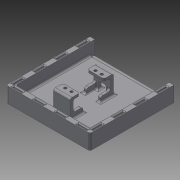
# Autodesk Inventor part: base_bottombuttonsBox
Saved by Autodesk Inventor 2014 (Build 180170000, 170)
## iProperties
Created: 2014-04-22
Part Number: base_bottombuttonsBox
Material: Generic
Document SubType Name: Modeling
Designer: t_emanb
Density: 1 g/cm^3
Appearance: Default
Author: t_emanb
Autodesk Inventor part; units mm, degrees
ref_plane "YZ Plane" through (0, 0, 0) normal (1, 0, 0) x (0, 1, 0)
ref_plane "XZ Plane" through (0, 0, 0) normal (0, 1, 0) x (-1, 0, 0)
ref_plane "XY Plane" through (0, 0, 0) normal (0, 0, 1) x (1, 0, 0)
sketch "Sketch1" plane through (0, 0, 0) normal (0, 1, 0) x (-1, 0, 0)
  line L0 (0, 0) -> (133.35, 0)
  line L1 (133.35, 0) -> (133.35, 133.35)
  line L2 (133.35, 133.35) -> (0, 133.35)
  line L3 (0, 133.35) -> (0, 0)
  dimension "d0" = 133.35
  dimension "d1" = 133.35
  constraints: 8 end point, 2 parallel, 1 horizontal, 1 perpendicular
  measures "d0" distance of L2.end L0.start
  measures "d1" distance of L0.start L0.end
extrude "Extrusion1" add sketch "Sketch1" along normal blind 5.08
sketch "Sketch2" plane through (0, 5.08, 0) normal (0, 1, 0) x (1, 0, 0)
  line L0 (0, 0) -> (-133.35, 0) projected
  line L1 (-133.35, 0) -> (-133.35, -133.35) projected
  line L2 (-133.35, -133.35) -> (0, -133.35) projected
  line L3 (0, -133.35) -> (0, 0) projected
  line L4 (-7.62, 0) -> (-7.62, -125.73)
  line L5 (-7.62, -125.73) -> (-125.73, -125.73)
  line L6 (-125.73, -125.73) -> (-125.73, 0)
  dimension "d4" = 7.62
  dimension "d5" = 7.62
  dimension "d6" = 7.62
  constraints: 6 end point, 2 point on line
  measures "d4" distance between parallel lines of L3 L4
  measures "d5" distance between parallel lines of L2 L5
  measures "d6" distance between parallel lines of L1 L6
extrude "Extrusion2" add sketch "Sketch2" along normal blind 19.05 contours L3 L2 L1 L0 L6 L5 L4
sketch "Sketch3" plane through (0, 24.13, 0) normal (0, 1, 0) x (1, 0, 0)
  line L0 (-7.62, -125.73) -> (-125.73, -125.73) projected
  line L1 (-125.73, -125.73) -> (-125.73, 0) projected
  line L2 (-133.35, 0) -> (-133.35, -133.35) projected
  line L3 (-133.35, -133.35) -> (0, -133.35) projected
  line L4 (-125.73, -130.81) -> (-110.49, -130.81)
  line L5 (-110.49, -130.81) -> (-110.49, -128.27)
  line L6 (-110.49, -128.27) -> (-125.73, -128.27)
  line L7 (-125.73, -128.27) -> (-125.73, -130.81)
  line L8 (-128.27, -125.73) -> (-130.81, -125.73)
  line L9 (-130.81, -125.73) -> (-130.81, -110.49)
  line L10 (-130.81, -110.49) -> (-128.27, -110.49)
  line L11 (-128.27, -110.49) -> (-128.27, -125.73)
  line L12 (-91.44, -130.81) -> (-76.2, -130.81)
  line L13 (-76.2, -130.81) -> (-76.2, -128.27)
  line L14 (-76.2, -128.27) -> (-91.44, -128.27)
  line L15 (-91.44, -128.27) -> (-91.44, -130.81)
  line L16 (-57.15, -130.81) -> (-41.91, -130.81)
  line L17 (-41.91, -130.81) -> (-41.91, -128.27)
  line L18 (-41.91, -128.27) -> (-57.15, -128.27)
  line L19 (-57.15, -128.27) -> (-57.15, -130.81)
  line L20 (-22.86, -130.81) -> (-7.62, -130.81)
  line L21 (-7.62, -130.81) -> (-7.62, -128.27)
  line L22 (-7.62, -128.27) -> (-22.86, -128.27)
  line L23 (-22.86, -128.27) -> (-22.86, -130.81)
  line L24 (-128.27, -91.44) -> (-130.81, -91.44)
  line L25 (-130.81, -91.44) -> (-130.81, -76.2)
  line L26 (-130.81, -76.2) -> (-128.27, -76.2)
  line L27 (-128.27, -76.2) -> (-128.27, -91.44)
  line L28 (-128.27, -57.15) -> (-130.81, -57.15)
  line L29 (-130.81, -57.15) -> (-130.81, -41.91)
  line L30 (-130.81, -41.91) -> (-128.27, -41.91)
  line L31 (-128.27, -41.91) -> (-128.27, -57.15)
  line L32 (-128.27, -22.86) -> (-130.81, -22.86)
  line L33 (-130.81, -22.86) -> (-130.81, -7.62)
  line L34 (-130.81, -7.62) -> (-128.27, -7.62)
  line L35 (-128.27, -7.62) -> (-128.27, -22.86)
  line L36 (-66.675, -133.35) -> (-66.675, 0) construction
  line L37 (-5.08, -125.73) -> (-2.54, -125.73)
  line L38 (-2.54, -125.73) -> (-2.54, -110.49)
  line L39 (-2.54, -110.49) -> (-5.08, -110.49)
  line L40 (-5.08, -110.49) -> (-5.08, -125.73)
  line L41 (-5.08, -91.44) -> (-2.54, -91.44)
  line L42 (-2.54, -91.44) -> (-2.54, -76.2)
  line L43 (-2.54, -76.2) -> (-5.08, -76.2)
  line L44 (-5.08, -76.2) -> (-5.08, -91.44)
  line L45 (-5.08, -57.15) -> (-2.54, -57.15)
  line L46 (-2.54, -57.15) -> (-2.54, -41.91)
  line L47 (-2.54, -41.91) -> (-5.08, -41.91)
  line L48 (-5.08, -41.91) -> (-5.08, -57.15)
  line L49 (-5.08, -22.86) -> (-2.54, -22.86)
  line L50 (-2.54, -22.86) -> (-2.54, -7.62)
  line L51 (-2.54, -7.62) -> (-5.08, -7.62)
  line L52 (-5.08, -7.62) -> (-5.08, -22.86)
  dimension "d9" = 15.24
  dimension "d10" = 15.24
  dimension "d11" = 2.54
  dimension "d12" = 2.54
  dimension "d13" = 2.54
  dimension "d14" = 2.54
  dimension "d17" = 34.29
  dimension "d24" = 34.29
  constraints: 98 end point, 16 symmetric about line, 5 parallel, 3 horizontal, 2 collinear, 2 perpendicular, 1 midpoint, 1 vertical, 48 other
  measures "d9" distance of L4.start L4.end
  measures "d10" distance of L8.end L9.end
  measures "d11" distance of L4.end L5.end
  measures "d12" distance of L9.end L10.end
  measures "d13" distance between parallel lines of L3 L4
  measures "d14" distance between parallel lines of L2 L9
  measures "d17" distance of L4.start L12.start
  measures "d24" distance of L8.start L24.start
extrude "Extrusion3" cut sketch "Sketch3" against normal blind 8.89
sketch "Sketch4" plane through (0, 0, 0) normal (0, 0, -1) x (-1, 0, 0)
  line L0 (0, 0) -> (133.35, 0) projected
  line L1 (7.62, 5.08) -> (125.73, 5.08) projected
  line L2 (0, 24.13) -> (7.62, 24.13) projected
  line L3 (0, 0) -> (0, 24.13) projected
  line L4 (2.54, 21.59) -> (5.08, 21.59)
  line L5 (5.08, 21.59) -> (5.08, 7.62)
  line L6 (5.08, 7.62) -> (2.54, 7.62)
  line L7 (2.54, 7.62) -> (2.54, 21.59)
  line L8 (7.62, 5.08) -> (7.62, 2.54)
  line L9 (7.62, 2.54) -> (125.73, 2.54)
  line L10 (125.73, 2.54) -> (125.73, 5.08)
  line L11 (66.675, 0) -> (66.675, 19.05) construction
  line L12 (130.81, 21.59) -> (128.27, 21.59)
  line L13 (128.27, 21.59) -> (128.27, 7.62)
  line L14 (128.27, 7.62) -> (130.81, 7.62)
  line L15 (130.81, 7.62) -> (130.81, 21.59)
  dimension "d31" = 2.54
  dimension "d32" = 13.97
  dimension "d33" = 2.54
  dimension "d34" = 2.54
  dimension "d35" = 2.54
  constraints: 24 end point, 5 parallel, 4 symmetric about line, 2 perpendicular, 1 horizontal, 1 midpoint
  measures "d31" distance of L4.start L4.end
  measures "d32" distance of L6.end L4.start
  measures "d33" distance between parallel lines of L3 L7
  measures "d34" distance between parallel lines of L2 L4
  measures "d35" distance between parallel lines of L1 L9
extrude "Extrusion4" cut sketch "Sketch4" against normal blind 6.35
fillet "Fillet1" radius 3.175 7 edges at (0, 12.065, 133.35) (-133.35, 12.065, 133.35) (-125.73, 5.08, 66.04) (-125.73, 14.605, 125.73) (-66.675, 5.08, 125.73) (-7.62, 14.605, 125.73) (-7.62, 5.08, 66.04)
sketch "Sketch5" plane through (0, 5.08, 0) normal (0, 1, 0) x (1, 0, 0)
  line L0 (-57.277, -96.266) -> (-76.073, -96.266) construction
  line L1 (-76.073, -96.266) -> (-76.073, -57.658) construction
  line L2 (-76.073, -57.658) -> (-57.277, -57.658) construction
  line L3 (-57.277, -57.658) -> (-57.277, -96.266) construction
  line L4 (-10.795, -125.73) -> (-122.555, -125.73) projected
  line L5 (-125.73, -122.555) -> (-125.73, 0) projected
  line L6 (-66.675, -96.266) -> (-66.675, -57.658) construction
  line L7 (-7.62, 0) -> (-7.62, -122.555) projected
  line L8 (-57.277, -47.498) -> (-76.073, -47.498)
  line L9 (-76.073, -47.498) -> (-76.073, -62.738)
  line L10 (-76.073, -62.738) -> (-79.883, -62.738)
  line L11 (-79.883, -62.738) -> (-79.883, -42.418)
  line L12 (-79.883, -42.418) -> (-53.467, -42.418)
  line L13 (-53.467, -42.418) -> (-53.467, -62.738)
  line L14 (-53.467, -62.738) -> (-57.277, -62.738)
  line L15 (-57.277, -62.738) -> (-57.277, -47.498)
  line L16 (-76.073, -76.962) -> (-57.277, -76.962) construction
  line L17 (-57.277, -106.426) -> (-76.073, -106.426)
  line L18 (-76.073, -106.426) -> (-76.073, -91.186)
  line L19 (-76.073, -91.186) -> (-79.883, -91.186)
  line L20 (-79.883, -91.186) -> (-79.883, -111.506)
  line L21 (-79.883, -111.506) -> (-53.467, -111.506)
  line L22 (-53.467, -111.506) -> (-53.467, -91.186)
  line L23 (-53.467, -91.186) -> (-57.277, -91.186)
  line L24 (-57.277, -91.186) -> (-57.277, -106.426)
  line L25 (-10.795, -122.555) -> (-122.555, -122.555) projected
  line L26 (-10.795, -6.35) -> (-122.555, -6.35) projected
  line L27 (-66.675, -6.35) -> (-66.675, -122.555) construction
  point P0 (0, 0)
  dimension "d42" = 29.464
  dimension "d44" = 38.608
  dimension "d64" = 18.796
  dimension "d71" = 10.16
  dimension "d74" = 5.08
  dimension "d75" = 5.08
  dimension "d76" = 3.81
  constraints: 46 end point, 8 symmetric about line, 6 perpendicular, 5 midpoint, 4 parallel, 2 point on line, 1 collinear, 1 horizontal, 3 other
  measures "d42" distance between parallel lines of L4 L0
  measures "d44" distance of L0.end L1.end
  measures "d64" distance between parallel lines of L3 L1
  measures "d71" distance between parallel lines of L8 L2
  measures "d74" distance between parallel lines of L12 L8
  measures "d75" distance between parallel lines of L14 L2
  measures "d76" distance of L13.end L14.end
extrude "Extrusion8" add sketch "Sketch5" along normal blind 7.9756
sketch "Sketch9" plane through (0, 13.0556, 0) normal (0, 1, 0) x (1, 0, 0)
  line L0 (-76.073, -47.498) -> (-57.277, -47.498) projected
  line L1 (-53.467, -62.738) -> (-53.467, -42.418) projected
  line L2 (-53.467, -42.418) -> (-79.883, -42.418) projected
  line L3 (-79.883, -42.418) -> (-79.883, -62.738) projected
  line L4 (-76.073, -106.426) -> (-76.073, -91.186) projected
  line L5 (-76.073, -91.186) -> (-79.883, -91.186) projected
  line L6 (-79.883, -91.186) -> (-79.883, -111.506) projected
  line L7 (-79.883, -111.506) -> (-53.467, -111.506) projected
  line L8 (-53.467, -111.506) -> (-53.467, -91.186) projected
  line L9 (-53.467, -91.186) -> (-57.277, -91.186) projected
  line L10 (-57.277, -91.186) -> (-57.277, -106.426) projected
  line L11 (-57.277, -106.426) -> (-76.073, -106.426) projected
  line L12 (-76.073, -47.498) -> (-79.883, -47.498)
  line L13 (-57.277, -47.498) -> (-53.467, -47.498)
  line L14 (-76.073, -106.426) -> (-79.883, -106.426)
  line L15 (-57.277, -106.426) -> (-53.467, -106.426)
  point P0 (0, 0)
  constraints: 8 end point, 4 point on line, 2 collinear, 2 perpendicular
extrude "Extrusion9" add sketch "Sketch9" along normal blind 17.78 contours L12 L3 L2 L1 L13 L0 | L11 L15 L8 L7 L6 L14
sketch "Sketch10" plane through (-53.467, 5.08, 111.506) normal (1, 0, 0) x (0, 0, -1)
  line L0 (20.32, 0) -> (0, 0) projected
  line L1 (0, 25.7556) -> (5.08, 25.7556) projected
  line L2 (69.088, 0) -> (48.768, 0) projected
  line L3 (69.088, 0) -> (69.088, 25.7556) projected
  line L4 (64.008, 25.7556) -> (69.088, 25.7556) projected
  line L5 (64.008, 7.9756) -> (64.008, 25.7556) projected
  line L6 (48.768, 7.9756) -> (64.008, 7.9756) projected
  line L7 (48.768, 0) -> (48.768, 7.9756) projected
  line L8 (0, 25.7556) -> (0, 29.5656)
  line L9 (0, 29.5656) -> (15.24, 29.5656)
  line L10 (15.24, 29.5656) -> (15.24, 25.7556)
  line L11 (15.24, 25.7556) -> (5.08, 25.7556)
  line L12 (69.088, 25.7556) -> (69.088, 29.5656)
  line L13 (69.088, 29.5656) -> (53.848, 29.5656)
  line L14 (53.848, 29.5656) -> (53.848, 25.7556)
  line L15 (53.848, 25.7556) -> (64.008, 25.7556)
  line L16 (5.08, 7.9756) -> (5.08, 25.7556) projected
  point P0 (111.506, -5.08)
  dimension "d81" = 3.81
  dimension "d95" = 10.16
  dimension "d96" = 10.16
  constraints: 16 end point, 5 parallel, 4 perpendicular, 1 collinear
  measures "d81" distance of L9.end L10.end
  measures "d95" distance between parallel lines of L10 L16
  measures "d96" distance between parallel lines of L5 L14
extrude "Extrusion10" add sketch "Sketch10" against normal up to surface (26.416 mm away) contours L8 L9 L10 L11 L1 | L4 L15 L14 L13 L12
sketch "Sketch11" plane through (-53.467, 34.6456, 111.506) normal (0, 1, 0) x (1, 0, 0)
  line L0 (0, 0) -> (-26.416, 0) projected
  line L1 (-26.416, 69.088) -> (-26.416, 53.848) projected
  line L2 (0, 53.848) -> (-26.416, 53.848) projected
  line L3 (0, 69.088) -> (0, 53.848) projected
  line L4 (0, 69.088) -> (-26.416, 69.088) projected
  line L5 (-13.208, 69.088) -> (-13.208, 0) construction
  line L6 (-13.208, 34.544) -> (-71.1791, 34.544) construction
  line L7 (-10.5156, 58.543) -> (-10.5156, 53.844) construction
  line L8 (-14.478, 58.924) -> (-14.478, 53.844)
  line L9 (-15.9004, 58.543) -> (-15.9004, 53.844) construction
  circle A0 centre (-8.2656, 58.543) radius 2.25
  circle A1 centre (-18.1504, 58.543) radius 2.25
  line L10 (-22.608, 53.844) -> (-3.808, 53.844)
  line L11 (-3.808, 34.544) -> (-22.608, 34.544) construction
  line L12 (-3.808, 53.844) -> (-3.808, 15.244)
  line L13 (-13.208, 48.0292) -> (-13.208, 10.164) construction
  line L14 (-22.608, 15.244) -> (-22.608, 53.844)
  arc A2 (-11.938, 58.924) -> (-14.478, 58.924) centre (-13.208, 58.924) ccw
  line L15 (-3.808, 15.244) -> (-22.608, 15.244)
  line L16 (-11.938, 53.844) -> (-11.938, 58.924)
  line L17 (-11.938, 10.164) -> (-11.938, 15.244)
  circle A3 centre (-8.2656, 10.545) radius 2.25
  arc A4 (-14.478, 10.164) -> (-11.938, 10.164) centre (-13.208, 10.164) ccw
  circle A5 centre (-18.1504, 10.545) radius 2.25
  line L18 (-14.478, 10.164) -> (-14.478, 15.244)
  point P0 (53.467, 111.506)
  dimension "d88" = 4.5
  dimension "d86" = 18.8
  dimension "d87" = 38.6
  dimension "d89" = 4.699
  dimension "d90" = 2.54
  dimension "d91" = 5.08
  dimension "d92" = 5.3848
  constraints: 28 end point, 7 point on line, 6 perpendicular, 6 symmetric about line, 5 midpoint, 4 centre point, 4 parallel, 4 point on circle, 3 tangent, 3 vertical, 2 coincident, 2 collinear, 2 horizontal alignment, 1 horizontal, 9 other
  measures "d86" distance of L15.start L15.end
  measures "d87" distance of L10.end L15.start
  measures "d89" distance from line of L10 point (-8.266, 58.543)
  measures "d90" distance between parallel lines of L16 L8
  measures "d91" distance from line of L10 A2.centre
  measures "d92" distance between parallel lines of L7 L9
extrude "Extrusion11" cut sketch "Sketch11" against normal up to surface (3.81 mm away) contours A0 | A1 | A3 | A5
sketch "Sketch12" plane through (-53.467, 5.08, 42.418) normal (0, 0, -1) x (-1, 0, 0)
  line L0 (26.416, 0) -> (0, 0) projected
  line L1 (0, 29.5656) -> (26.416, 29.5656) projected
  line L2 (6.858, 0) -> (19.558, 0)
  line L3 (19.558, 0) -> (19.558, 9.525)
  line L4 (16.383, 12.7) -> (10.033, 12.7)
  line L5 (6.858, 9.525) -> (6.858, 0)
  line L6 (13.208, 29.5656) -> (13.208, 0) construction
  arc A0 (10.033, 12.7) -> (6.858, 9.525) centre (10.033, 9.525) ccw
  arc A1 (19.558, 9.525) -> (16.383, 12.7) centre (16.383, 9.525) ccw
  point P0 (-53.467, -5.08)
  point P1 (19.558, 12.7)
  point P2 (6.858, 12.7)
  dimension "d97" = 12.7
  dimension "d98" = 12.7
  dimension "d99" = 3.175
  constraints: 10 end point, 5 point on line, 4 point on circle, 4 tangent, 2 centre point, 2 midpoint, 2 parallel, 2 perpendicular, 1 equal radius, 1 horizontal, 1 other
  measures "d97" distance between parallel lines of L0 L4
  measures "d98" distance of point (19.558, 12.7) point (6.858, 12.7)
  measures "d99" radius of A0
extrude "Extrusion12" cut sketch "Sketch12" against normal up to surface (5.08 mm away)
fillet "Fillet2" radius 3.175 32 edges at (-73.025, 5.08, 44.958) (-74.549, 5.08, 47.498) (-77.978, 5.08, 62.738) (-79.883, 5.08, 52.578) (-76.454, 5.08, 42.418) (-56.896, 5.08, 42.418) (-53.467, 5.08, 52.578) (-55.372, 5.08, 62.738) (-58.801, 5.08, 47.498) (-60.325, 5.08, 44.958) (-66.675, 5.08, 106.426) (-55.372, 5.08, 91.186) (-53.467, 5.08, 101.346) (-66.675, 5.08, 111.506) (-79.883, 5.08, 101.346) (-77.978, 5.08, 91.186) (-66.675, 34.6456, 42.418) (-66.675, 30.8356, 47.498) (-66.675, 34.6456, 111.506) (-66.675, 30.8356, 106.426) (-77.978, 13.0556, 47.498) (-55.372, 13.0556, 47.498) (-77.978, 13.0556, 106.426) (-55.372, 13.0556, 106.426) (-55.372, 13.0556, 91.186) (-77.978, 13.0556, 91.186) (-77.978, 13.0556, 62.738) (-55.372, 13.0556, 62.738) (-79.883, 32.7406, 57.658) (-53.467, 32.7406, 57.658) (-79.883, 32.7406, 96.266) (-53.467, 32.7406, 96.266)
fillet "Fillet3" radius 3.175 4 edges at (-3.81, 7.62, 0) (-3.81, 21.59, 0) (-129.54, 7.62, 0) (-129.54, 21.59, 0)
fillet "Fillet4" radius 1.27 21 edges at (-66.675, 2.54, 6.35) (-66.675, 2.54, 0) (-124.8001, 6.0099, 6.35) (-8.5499, 6.0099, 6.35) (-66.675, 5.08, 6.35) (-57.277, 6.0099, 48.4279) (-57.277, 12.2428, 47.498) (-57.277, 5.08, 58.293) (-76.073, 6.0099, 48.4279) (-76.073, 12.2428, 47.498) (-76.073, 5.08, 58.293) (-57.277, 6.0099, 105.4961) (-57.277, 12.2428, 106.426) (-57.277, 5.08, 95.631) (-76.073, 6.0099, 105.4961) (-76.073, 12.2428, 106.426) (-76.073, 5.08, 95.631) (-3.81, 21.59, 6.35) (-3.81, 7.62, 6.35) (-129.54, 7.62, 6.35) (-129.54, 21.59, 6.35)
fillet "Fillet5" radius 2.54 24 edges at (-3.81, 15.24, 7.62) (-3.81, 15.24, 22.86) (-3.81, 15.24, 41.91) (-3.81, 15.24, 57.15) (-3.81, 15.24, 91.44) (-3.81, 15.24, 76.2) (-3.81, 15.24, 110.49) (-3.81, 15.24, 125.73) (-7.62, 15.24, 129.54) (-22.86, 15.24, 129.54) (-41.91, 15.24, 129.54) (-57.15, 15.24, 129.54) (-76.2, 15.24, 129.54) (-91.44, 15.24, 129.54) (-110.49, 15.24, 129.54) (-125.73, 15.24, 129.54) (-129.54, 15.24, 125.73) (-129.54, 15.24, 110.49) (-129.54, 15.24, 91.44) (-129.54, 15.24, 76.2) (-129.54, 15.24, 57.15) (-129.54, 15.24, 41.91) (-129.54, 15.24, 22.86) (-129.54, 15.24, 7.62)
fillet "Fillet6" radius 1.524 48 edges at (-128.27, 24.13, 15.24) (-129.54, 24.13, 22.86) (-130.81, 24.13, 15.24) (-129.54, 24.13, 7.62) (-128.27, 24.13, 49.53) (-129.54, 24.13, 57.15) (-130.81, 24.13, 49.53) (-129.54, 24.13, 41.91) (-128.27, 24.13, 83.82) (-129.54, 24.13, 91.44) (-130.81, 24.13, 83.82) (-129.54, 24.13, 76.2) (-128.27, 24.13, 118.11) (-129.54, 24.13, 125.73) (-130.81, 24.13, 118.11) (-129.54, 24.13, 110.49) (-110.49, 24.13, 129.54) (-118.11, 24.13, 130.81) (-125.73, 24.13, 129.54) (-118.11, 24.13, 128.27) (-76.2, 24.13, 129.54) (-83.82, 24.13, 130.81) (-91.44, 24.13, 129.54) (-83.82, 24.13, 128.27) (-41.91, 24.13, 129.54) (-49.53, 24.13, 130.81) (-57.15, 24.13, 129.54) (-49.53, 24.13, 128.27) (-7.62, 24.13, 129.54) (-15.24, 24.13, 130.81) (-22.86, 24.13, 129.54) (-15.24, 24.13, 128.27) (-2.54, 24.13, 118.11) (-3.81, 24.13, 125.73) (-5.08, 24.13, 118.11) (-3.81, 24.13, 110.49) (-5.08, 24.13, 83.82) (-3.81, 24.13, 76.2) (-2.54, 24.13, 83.82) (-3.81, 24.13, 91.44) (-2.54, 24.13, 49.53) (-3.81, 24.13, 57.15) (-5.08, 24.13, 49.53) (-3.81, 24.13, 41.91) (-2.54, 24.13, 15.24) (-3.81, 24.13, 22.86) (-5.08, 24.13, 15.24) (-3.81, 24.13, 7.62)
equation "\"d5\" = d4"
equation "\"d6\" = d4"
equation "\"d10\" = d9"
equation "\"d12\" = d11"
equation "\"d14\" = d13"
body "Solid1"
